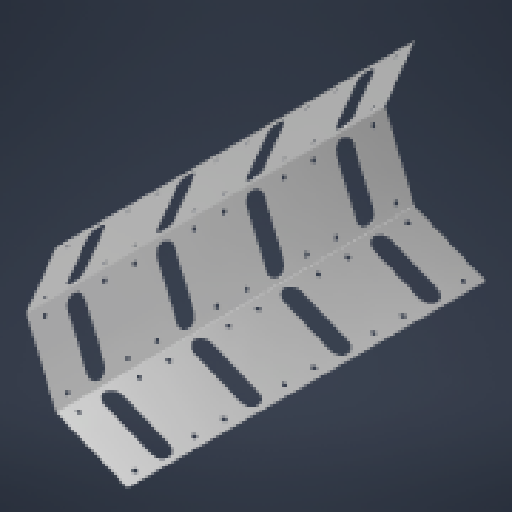
# Autodesk Inventor part: DMF 01 13 Барабан Лист лев брт v2.1
Saved by Autodesk Inventor 2026.2 (Build 302298010, 298A)
## iProperties
Created: 2024-04-28
Part Number: DMF 01 13 Барабан Лист лев брт v2.1
Material: Stainless Steel AISI 304
Document SubType Name: Sheet Metal
Designer: pokla
Density: 8 g/cm^3
Appearance: Chrome - Satin
Sheet Metal Rule: Default
Flat Pattern Width: 63.6056 cm
Flat Pattern Length: 98.3 cm
Flat Pattern Area: 6252.43 cm^2
Sheet Metal Width: 636,056 mm
Sheet Metal Length: 983,000 mm
Sheet Metal Area: 625243,471 mm^2
Stock Number: Барабан_Лист_Левый_Борт
d218: 145,000 mm
d219: 50,000 mm
d228: 145,000 mm
d229: 50,000 mm
Author: pokla
Autodesk Inventor part; units mm, degrees
note: some values were not read from the file. Chosen so that the rebuilt part matches the saved one: flange form of "Plate6"; pattern direction of "Circular Pattern3".
ref_plane "YZ Plane" through (0, 0, 0) normal (1, 0, 0) x (0, 1, 0)
ref_plane "XZ Plane" through (0, 0, 0) normal (0, 1, 0) x (-1, 0, 0)
ref_plane "XY Plane" through (0, 0, 0) normal (0, 0, 1) x (1, 0, 0)
sketch "Sketch2" plane through (0, 0, 0) normal (0, 0, 1) x (1, 0, 0)
  line L0 (0, 278.716) -> (197.082, 197.082) construction
  line L1 (197.082, 197.082) -> (278.716, 0) construction
  line L2 (278.716, 0) -> (197.082, -197.082) construction
  line L3 (197.082, -197.082) -> (0, -278.716) construction
  line L4 (0, -278.716) -> (-197.082, -197.082) construction
  line L5 (-197.082, -197.082) -> (-278.716, 0) construction
  line L6 (-278.716, 0) -> (-197.082, 197.082) construction
  line L7 (-197.082, 197.082) -> (0, 278.716) construction
  line L8 (-278.0819, -1.5307) -> (-197.716, -195.5512)
  line L9 (-195.5512, -197.716) -> (-0.8315, -278.3716)
  arc A0 (-278.0819, 1.5307) -> (-278.0819, -1.5307) centre (-274.3864, 0) ccw
  arc A1 (-197.716, -195.5512) -> (-195.5512, -197.716) centre (-194.0205, -194.0205) ccw
  line L10 (-278.0819, 1.5307) -> (-197.4264, 196.2505)
  point P0 (0, 0)
  point P1 (0, 0)
  dimension "d58" = 4
  dimension "d59" = 4
  dimension "d70" = 0.9
  dimension "d72" = 0.9
  dimension "d74" = 515
  measures "d58" radius of A0
  measures "d59" radius of A1
  measures "d70" distance of L3.end L9.end
  measures "d72" distance of L6.end L10.end
  measures "d74" distance between parallel lines of L1 L8
contour flange "Contour Flange3" sketch "Sketch2" thickness 2 bend radius 2 width 983 along (0, 0, -1) mid plane no both sides no wall seen from (-98.1914, -238.0438, 0) lies toward (0.3826834, 0.9238795, 0) curves L9 A1 L8 A0 L10
bend "Bend6"
corner "Corner6"
sketch "Sketch15" plane through (-278.0819, -1.5307, -983) normal (-0.9238795, -0.3826834, 0) x (0, 0, 1)
  line L0 (0, -210.0063) -> (0, 0) projected
  line L1 (983, -210.0063) -> (983, 0) projected
  line L2 (835, -36.5031) -> (885, -36.5031)
  line L3 (885, -36.5031) -> (885, -173.5031)
  line L4 (885, -173.5031) -> (835, -173.5031)
  line L5 (835, -173.5031) -> (835, -36.5031)
  line L6 (835, -36.5031) -> (885, -173.5031) construction
  line L7 (885, -36.5031) -> (835, -173.5031) construction
  arc A0 (885, -36.5031) -> (835, -36.5031) centre (860, -36.5031) ccw
  arc A1 (835, -173.5031) -> (885, -173.5031) centre (860, -173.5031) ccw
  circle A2 centre (777.5, -22.5031) radius 5.5
  circle A3 centre (942.5, -22.5031) radius 5.5
  line L8 (860, -36.5031) -> (860, -173.5031) construction
  line L9 (885, -105.0031) -> (835, -105.0031) construction
  circle A4 centre (777.5, -187.5031) radius 5.5
  circle A5 centre (942.5, -187.5031) radius 5.5
  circle A6 centre (777.5, -22.5031) radius 6.5
  circle A7 centre (860, -22.5031) radius 6.5
  circle A8 centre (860, -187.5031) radius 6.5
  circle A9 centre (777.5, -187.5031) radius 6.5
  circle A10 centre (942.5, -187.5031) radius 6.5
  circle A11 centre (942.5, -22.5031) radius 6.5
  point P0 (0, -105.0031)
  point P1 (860, -105.0031)
  point P2 (860, -105.0031)
  point P3 (983, -105.0031)
  dimension "d220" = 137
  dimension "d221" = 50
  dimension "d222" = 165
  dimension "d223" = 165
  dimension "d224" = 11
  dimension "d225" = 13
  dimension "d226" = 13
  dimension "d227" = 165
  dimension "d230" = 98
  constraints: 16 end point, 12 centre point, 7 midpoint, 4 coincident, 4 point on circle, 4 tangent, 3 equal radius, 2 parallel, 2 point on line, 1 horizontal, 1 horizontal alignment, 1 perpendicular, 1 vertical, 4 other
  measures "d220" distance of L2.end L3.end
  measures "d221" distance of L2.start L2.end
  measures "d222" distance of A3.centre A2.centre
  measures "d223" distance of A5.centre A3.centre
  measures "d224" diameter of A2
  measures "d225" diameter of A6
  measures "d226" diameter of A7
  measures "d227" distance of A8.centre A7.centre
  measures "d230" distance between parallel lines of L1 L3
extrude "Cut1" cut sketch "Sketch15" against normal through all contours A0 L2 | L2 L3 L4 L5 | L4 A1 | A2 | A3 | A4 | A5 | A6 | A7 | A8 | A9 | A10 | A11
pattern_linear "Rectangular Pattern3" count 4 spacing 246 along (0, 0, -1) of "Cut1"
pattern_circular "Circular Pattern3" count 3 over 90 about axis through (0, 0, -10) along (0, 0, 1) of "Cut1", "Rectangular Pattern3" both ways yes
equation "\"d58\" = BendRadius + Thickness"
equation "\"d59\" = BendRadius + Thickness"
equation "\"d74\" = Барабан_размер_по_плоскостям"
equation "\"d75\" = Thickness"
equation "\"d76\" = BendReliefWidth"
equation "\"d77\" = BendReliefDepth"
equation "\"d78\" = MinimumRemnant"
equation "\"d79\" = TransitionRadius"
equation "\"d81\" = BendRadius"
equation "\"d83\" = CornerReliefSize"
equation "\"d84\" = GapSize"
equation "\"d85\" = JacobiRadiusSize"
equation "\"BendRadius\" = Thickness"
equation "\"BendReliefWidth\" = Thickness"
equation "\"BendReliefDepth\" = 0.5 * Thickness"
equation "\"CornerReliefSize\" = 4 * Thickness"
equation "\"MinimumRemnant\" = 2 * Thickness"
equation "\"TransitionRadius\" = BendRadius"
equation "\"JacobiRadiusSize\" = BendRadius"
equation "\"GapSize\" = Thickness"
equation "\"Барабан_Середина_листа\" = 206.27835"
equation "\"d218\" = 145"
equation "\"d228\" = 145"
equation "\"Thickness\" = 2"
equation "\"Барабан_размер_по_плоскостям\" = 515"
body "Solid3"
